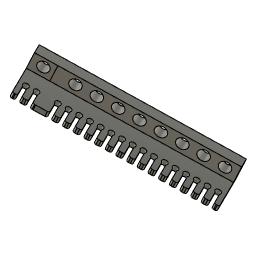
LED90Degree v16 (Autodesk Fusion 360 design; units mm, degrees)
Autodesk Fusion 360 part; units mm, degrees
note: some values were not read from the file. Set by a fixed rule: which sketch regions a step uses.
sketch "LEDHoleBarProfile" plane through (0, 0, 0) normal (0, 1, 0) x (1, 0, 0)
  line L0 (0, 0) -> (5.08, 0)
  line L1 (5.08, 0) -> (5.08, -3)
  line L2 (5.08, -3) -> (0, -3)
  line L3 (0, -3) -> (0, 0)
  dimension "d1" = 5.08
  dimension "d2" = 3
  constraint horizontal L0
  constraint vertical L1
  constraint horizontal L2
  constraint vertical L3
  constraint coincident L0.start L3.end
  measures "d1" distance of L0.start L0.end
  measures "d2" distance of L0.start L2.end
extrude "Extrude1" add sketch "LEDHoleBarProfile" along normal blind 3.75 makes body 1
sketch "LEDHolePosition" plane through (0, 0, 3) normal (0, 0, 1) x (1, 0, 0)
  line L0 (0, 0) -> (5.08, 0)
  line L1 (5.08, 0) -> (5.08, 3.75)
  line L2 (5.08, 3.75) -> (0, 3.75)
  line L3 (0, 3.75) -> (0, 0)
  circle A0 centre (2.54, 1.75) radius 1.505
  dimension "d5" = 3.01
  dimension "d7" = 2.54
  dimension "d8" = 2.25
  dimension "d9" = 2
  dimension "d10" = 2
  measures "d5" diameter of A0
  measures "d7" distance of L1 A0.centre
  measures "d9" distance of L2 A0.centre
extrude "Extrude2" cut sketch "LEDHolePosition" against normal blind 3 contours A0 bodies 1
extrude "Extrude3" add 1 faces at (1.6933, 3.75, 1) along direction (0, 1, 0) blind 2 on bodies 1 bodies 1
sketch "BaseSegment" plane through (0, 0, 3) normal (0, 0, 1) x (1, 0, 0)
  circle A0 centre (2.54, 1.75) radius 1.505
  line L0 (0, 0) -> (5.08, 0)
  line L1 (5.08, 0) -> (5.08, 5.75)
  line L2 (5.08, 5.75) -> (0, 5.75)
  line L3 (0, 5.75) -> (0, 0)
  line L4 (0, 5.75) -> (5.08, 5.75)
  line L5 (5.08, 5.75) -> (5.08, 4.25)
  line L6 (5.08, 4.25) -> (0, 4.25)
  line L7 (0, 4.25) -> (0, 5.75)
  dimension "d15" = 1.5
  dimension "d36" = 5.08
  constraint horizontal L4
  constraint vertical L5
  constraint horizontal L6
  constraint vertical L7
  constraint coincident L2.end L3.start
  measures "d15" distance of L2.end L6.end
  measures "d36" distance of L5 L7
extrude "Extrude4" add sketch "BaseSegment" along normal blind 9 contours L1 L2 L3 L4 L5 L6 L7 bodies 1
sketch "Wire Accomodations" plane through (0, 4.25, 0) normal (0, -1, 0) x (1, 0, 0)
  line L0 (0, 3) -> (5.08, 3)
  line L1 (5.08, 3) -> (5.08, 12)
  line L2 (5.08, 12) -> (0, 12)
  line L3 (0, 12) -> (0, 3)
  circle A0 centre (1.27, 8) radius 0.75
  circle A1 centre (3.81, 8) radius 0.75
  line L4 (3.33, 8) -> (4.33, 8)
  line L5 (4.33, 8) -> (4.33, 12)
  line L6 (4.33, 12) -> (3.33, 12)
  line L7 (3.33, 12) -> (3.33, 8)
  line L8 (1.75, 8) -> (0.75, 8)
  line L9 (0.75, 8) -> (0.75, 12)
  line L10 (0.75, 12) -> (1.75, 12)
  line L11 (1.75, 12) -> (1.75, 8)
  line L12 (0, 0) -> (5.08, 0)
  dimension "d18" = 1.5
  dimension "d19" = 1.5
  dimension "d23" = 2.54
  dimension "d24" = 1.27
  dimension "d25" = 2
  dimension "d30" = 4
  dimension "d31" = 4
  dimension "d38" = 1
  dimension "d39" = 4
  dimension "d40" = 1
  dimension "d41" = 4
  dimension "d44" = 9
  dimension "d45" = 9
  dimension "d46" = 3
  dimension "d47" = 0.75
  dimension "d48" = 0.75
  constraint horizontal L4
  constraint vertical L5
  constraint horizontal L6
  constraint vertical L7
  constraint horizontal L8
  constraint vertical L9
  constraint horizontal L10
  constraint vertical L11
  measures "d18" diameter of A0
  measures "d19" diameter of A1
  measures "d23" horizontal distance of A0.centre A1.centre
  measures "d24" distance of L1 A1.centre
  measures "d30" distance of L2 A0.centre
  measures "d31" distance of L2 A1.centre
  measures "d38" distance of L4.start L4.end
  measures "d39" distance of L4.start L6.end
  measures "d40" distance of L8.start L8.end
  measures "d41" distance of L8.start L10.end
  measures "d44" distance of L0 L6
  measures "d45" distance of L0 L10
  measures "d46" distance of L0 L12
  measures "d47" distance of L3 L9
  measures "d48" distance of L1 L5
extrude "Extrude9" cut sketch "Wire Accomodations" against normal blind 1.5 contours L2 A0 L9 L10 L11 | L2 A1 L5 L6 L7 bodies 1
fillet "Fillet1" radius 0.5 4 edges at (3.33, 5, 12) (4.33, 5, 12) (1.75, 5, 12) (0.75, 5, 12) on bodies 1
extrude "Extrude5" cut sketch "Wire Accomodations" against normal blind 1.5 contours A0 L8 L9 L11 | A0 L8 L9 L11 | A1 L4 L5 L7 | A1 L4 L5 L7 bodies 1
copy_body "CopyPasteBodies1" bodies 1 makes body 2
move_body "Move1" bodies 2 to x (1, 0, 0) y (0, 1, 0) z (0, 0, 1) at (5.08, 0, 0)
copy_body "CopyPasteBodies2" bodies 2 1 makes body 3 makes body 4
move_body "Move2" bodies 3 4 to x (1, 0, 0) y (0, 1, 0) z (0, 0, 1) at (10.16, 0, 0)
copy_body "CopyPasteBodies3" bodies 1 2 3 4 makes body 5 makes body 6 makes body 7 makes body 8
move_body "Move3" bodies 5 6 7 8 to x (1, 0, 0) y (0, 1, 0) z (0, 0, 1) at (20.32, 0, 0)
move_face "OffsetFaces1" offset 2.54 1 faces at (40.64, 3.3333, 1) on bodies 7
copy_body "CopyPasteBodies5" bodies 1 makes body 9
move_body "Move5" bodies 9 to x (1, 0, 0) y (0, 1, 0) z (0, 0, 1) at (43.1756, 0, -0.0001)
combine "Combine2" operation add target body 7 tool bodies 1 5 3 2 4 6 8 9
move_face "OffsetFaces2" offset 0.5 1 faces at (0, 3.3333, 1) on bodies 7
fillet "Fillet2" radius 0.5 1 edges at (-0.5, 5, 12) on bodies 7
move_face "OffsetFaces3" offset 0.5 1 faces at (48.2556, 3.3333, 0.9999) on bodies 7
fillet "Fillet3" radius 0.5 1 edges at (48.7556, 5, 11.9999) on bodies 7
move_face "OffsetFaces4" offset 0.5 1 faces at (28.6185, 0, 2) on bodies 7
equation "d24 = ( 2.54 / 2 ) * 1 mm"
